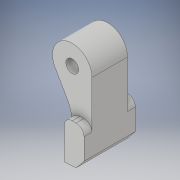
# Autodesk Inventor part: Fangklinke
Saved by Autodesk Inventor 2019 (Build 230136000, 136)
## iProperties
Created: 2021-03-08
Part Number: Fangklinke
Material: Generic
Document SubType Name: Modeling
Designer: Lukas
Density: 1 g/cm^3
Appearance: Default
Author: Lukas
Autodesk Inventor part; units mm, degrees
ref_plane "YZ Plane" through (0, 0, 0) normal (1, 0, 0) x (0, 1, 0)
ref_plane "XZ Plane" through (0, 0, 0) normal (0, 1, 0) x (-1, 0, 0)
ref_plane "XY Plane" through (0, 0, 0) normal (0, 0, 1) x (1, 0, 0)
sketch "Sketch1" plane through (0, 0, 0) normal (0, 0, 1) x (1, 0, 0)
  circle A0 centre (0, 0) radius 5
  circle A1 centre (0, 0) radius 1.6
  line L0 (-4.3301, -2.5) -> (0, -10)
  line L1 (0, -10) -> (0, -20)
  line L2 (5, -19.3649) -> (5, 0)
  arc A2 (0, -20) -> (5, -19.3649) centre (0, 0) ccw
  dimension "d0" = 10
  dimension "d1" = 3.2
  dimension "d2" = 5
  dimension "d3" = 10
  dimension "d5" = 10
  constraints: 6 end point, 4 point on circle, 3 centre point, 3 coincident, 2 tangent, 1 parallel, 1 vertical
  measures "d0" diameter of A0
  measures "d1" diameter of A1
  measures "d2" distance between parallel lines of L2 L1
  measures "d3" distance of point (0, 0) L0.end
  measures "d5" distance of L0.end L1.end
extrude "Extrusion1" add sketch "Sketch1" along normal blind 9
fillet "Fillet1" radius 10 1 edges at (0, -10, 4.5)
sketch "Sketch2" plane through (0, 0, 0) normal (0, 0, -1) x (-1, 0, 0)
  circle A0 centre (0, 0) radius 1.6 projected
  arc A1 (4.3301, -2.5) -> (-5, 0) centre (0, 0) ccw projected
  line L0 (-5, -19.3649) -> (-5, 0) projected
  line L1 (0, -12.6795) -> (0, -20) projected
  line L2 (4.3301, -2.5) -> (1.3397, -7.6795) projected
  line L3 (0, -10) -> (0, -20) projected
  line L4 (0, -10) -> (-5, -10)
  line L5 (0, -20) -> (-5, -19.5626) projected
  arc A2 (1.3397, -7.6795) -> (0, -12.6795) centre (10, -12.6795) ccw projected
  arc A3 (-5, -19.3649) -> (0, -20) centre (0, 0) ccw projected
  dimension "d8" = 10
  constraints: 2 end point, 2 point on line, 1 perpendicular
  measures "d8" distance from line of L1.end L4
extrude "Extrusion2" add sketch "Sketch2" along normal blind 2 and the other way blind 11 contours L4 L3 L1 L5 A3 L0 | A3 L5
chamfer "Chamfer1" distance 2 angle 45 3 edges at (5, -19.3649, -1) (5, -19.3649, 4.5) (5, -19.3649, 10)
sketch "Sketch3" plane through (0, 0, 9) normal (0, 0, -1) x (-1, 0, 0)
  circle A0 centre (-2.5, -15) radius 1.5
  line L0 (0, -10) -> (-5, -10) projected
  point P0 (0, 0)
  point P1 (-2.5, -10)
  dimension "d18" = 3
  dimension "d19" = 5
  constraints: 1 centre point, 1 midpoint, 1 vertical alignment
  measures "d18" diameter of A0
  measures "d19" distance from line of A0.centre L0
extrude "Extrusion3" cut sketch "Sketch3" along normal through all
fillet "Fillet2" radius 2 4 edges at (0, -10, -1) (5, -10, -1) (5, -10, 10) (0, -10, 10)
body "Solid1"
